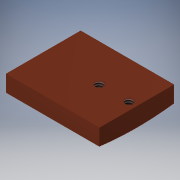
# Autodesk Inventor part: 4K adapter
Saved by Autodesk Inventor 2018 (Build 220112000, 112)
## iProperties
Created: 2019-03-13
Part Number: 4K adapter
Material: Copper
Document SubType Name: Modeling
Designer: Admin
Density: 8.94 g/cm^3
Appearance: Copper - Satin
Author: Admin
Autodesk Inventor part; units mm, degrees
ref_plane "YZ Plane" through (0, 0, 0) normal (1, 0, 0) x (0, 1, 0)
ref_plane "XZ Plane" through (0, 0, 0) normal (0, 1, 0) x (-1, 0, 0)
ref_plane "XY Plane" through (0, 0, 0) normal (0, 0, 1) x (1, 0, 0)
sketch "Sketch1" plane through (0, 0, 0) normal (0, 1, 0) x (-1, 0, 0)
  line L0 (-15.875, 12.7) -> (15.875, 12.7)
  line L1 (15.875, 12.7) -> (15.875, -12.7)
  line L2 (15.875, -12.7) -> (-15.875, -12.7)
  line L3 (-15.875, -12.7) -> (-15.875, 12.7)
  line L4 (-15.875, 12.7) -> (15.875, -12.7) construction
  line L5 (15.875, 12.7) -> (-15.875, -12.7) construction
  point P0 (0, 0)
  dimension "d0" = 31.75
  dimension "d1" = 25.4
  constraints: 12 end point, 2 midpoint, 2 parallel, 1 horizontal, 1 perpendicular
  measures "d0" distance of L1.end L2.end
  measures "d1" distance of L0.end L1.end
extrude "Extrusion1" add sketch "Sketch1" along normal blind 6.35
sketch "Sketch2" plane through (-15.875, 0, -12.7) normal (-1, 0, 0) x (0, 0, 1)
  line L0 (12.7, 0) -> (12.7, 6.35) construction
  line L1 (25.4, 6.35) -> (0, 6.35) construction
  line L2 (12.7, 3.175) -> (6.35, 3.175) construction
  line L3 (12.7, 3.175) -> (19.05, 3.175) construction
  dimension "d4" = 6.35
  dimension "d5" = 180
  constraints: 6 end point, 2 horizontal, 2 midpoint, 1 coincident, 1 collinear, 1 symmetric about line
  measures "d4" distance of L2.start L2.end
  measures "d5" angle of L2 L3
hole "Hole1" at (-15.875, 3.175, -6.35) at (-15.875, 3.175, 6.35) direction (1, 0, 0) diameter 2.6416 depth 19.05 tip angle 118 thread size "6-32 UNC" class "2B" standard "ANSI Unified Screw Threads"
sketch "Sketch3" plane through (-15.875, 0, -12.7) normal (-1, 0, 0) x (0, 0, 1)
  line L0 (12.7, 0) -> (12.7, 98.425) construction
  line L1 (12.7, 0) -> (111.125, 0) construction
  circle A0 centre (12.7, 98.425) radius 98.425
  dimension "d14" = 98.425
  dimension "d15" = 90
  dimension "d16" = 196.85
  constraints: 4 end point, 2 coincident, 1 centre point, 1 horizontal, 1 perpendicular, 1 vertical
  measures "d14" distance of L0.start L0.end
  measures "d15" angle of L1 L0
  measures "d16" diameter of A0
extrude "Extrusion2" cut sketch "Sketch3" against normal up to surface (31.75 mm away) keep common part
sketch "Sketch4" plane through (0, 6.35, 0) normal (0, 1, 0) x (1, 0, 0)
  line L0 (-15.875, 12.7) -> (-15.875, -12.7) construction
  line L1 (-15.875, 0) -> (3.175, 0) construction
  line L2 (-15.875, 0) -> (3.175, 0) construction
  line L3 (3.175, 0) -> (13.335, 0) construction
  line L4 (3.175, 0) -> (13.335, 0) construction
  point P0 (0, 0)
  dimension "d19" = 19.05
  dimension "d20" = 0
  dimension "d21" = 10.16
  dimension "d22" = 0
  constraints: 8 end point, 4 horizontal, 2 coincident, 2 collinear, 1 midpoint
  measures "d19" distance of L1.start L1.end
  measures "d20" distance between parallel lines of L1 L2
  measures "d21" distance of L2.end L3.end
  measures "d22" distance between parallel lines of L3 L4
hole "Hole2" at (13.335, 6.35, 0) at (3.175, 6.35, 0) direction (0, -1, 0) diameter 2.6416 depth 19.05 tip angle 118 thread size "6-32 UNC" class "2B" standard "ANSI Unified Screw Threads"
body "Solid1"
